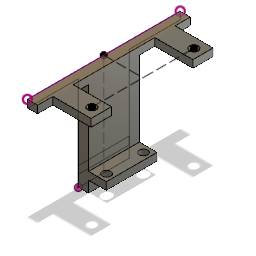
support_carte_front (Autodesk Fusion 360 design; units mm, degrees)
Autodesk Fusion 360 part; units mm, degrees
sketch "Sketch1" plane through (0, 0, 0) normal (1, 0, 0) x (0, 0, -1)
  line L0 (0, 0) -> (0, 37)
  line L1 (0, 37) -> (-20, 37)
  line L2 (-20, 37) -> (-20, 40)
  line L3 (-20, 40) -> (40, 40)
  line L4 (40, 40) -> (40, 37)
  line L5 (40, 37) -> (20, 37)
  line L6 (20, 37) -> (20, 0)
  line L7 (20, 0) -> (0, 0)
  line L8 (0, 4.5) -> (20, 4.5)
  line L9 (20, 4.5) -> (20, 7.5)
  line L10 (20, 7.5) -> (0, 7.5)
  line L11 (0, 7.5) -> (0, 4.5)
  line L12 (10, 0) -> (10, 40) construction
  point P0 (10, 40)
  dimension "d1" = 20
  dimension "d2" = 4.5
  dimension "d3" = 3
  dimension "d5" = 40
  dimension "d7" = 3
  dimension "d8" = 60
  constraint coincident L0.start L7.end
  constraint vertical L0
  constraint perpendicular L0 L1
  constraint perpendicular L1 L2
  constraint perpendicular L2 L3
  constraint perpendicular L3 L4
  constraint perpendicular L4 L5
  constraint perpendicular L3 L6
  constraint perpendicular L0 L7
  constraint horizontal L8
  constraint vertical L9
  constraint horizontal L10
  constraint vertical L11
  constraint coincident L6 L9.end
  constraint coincident L0 L8.start
  constraint collinear L1 L5
  constraint midpoint L3 P0
  constraint midpoint L7 L12.start
  constraint coincident L3 P0
  constraint perpendicular L3 L12
  constraint coincident P0 L12.end
  measures "d1" distance of L0 L6
  measures "d2" distance of L7 L8
  measures "d3" distance of L8 L10
  measures "d5" distance of L3 L7
  measures "d7" distance of L3 L5
  measures "d8" distance of L2 L4
  measures "d23" distance of L0.start
extrude "Extrude1" add sketch "Sketch1" along normal blind 4 makes body 1
extrude "Extrude2" add sketch "Sketch1" along normal blind 11 separate body contours L0 L6 L8 L9 L10 L11 makes body 2
sketch "Sketch2" plane through (0, 7.5, 0) normal (0, 1, 0) x (-1, 0, 0)
  line L0 (0, -20) -> (0, 0)
  line L1 (0, 0) -> (-11, 0)
  line L2 (-11, 0) -> (-11, -20)
  line L3 (-11, -20) -> (0, -20)
  circle A0 centre (-8.35, -17.25) radius 1.65
  circle A1 centre (-8.35, -2.75) radius 1.65
  line L4 (-8.35, -2.75) -> (-8.35, -17.25) construction
  line L5 (-11, -10) -> (-5.7, -10) construction
  point P0 (-8.35, -10)
  dimension "d15" = 14.5
  dimension "d16" = 2.65
  dimension "d17" = 3.3
  dimension "d18" = 3.3
  constraint coincident A1.centre L4.start
  constraint coincident A0.centre L4.end
  constraint parallel L0 L4
  constraint midpoint L2 L5.start
  constraint perpendicular L2 L5
  constraint midpoint L4 P0
  constraint midpoint L5 P0
  measures "d15" distance of A0.centre A1.centre
  measures "d16" distance of L2 L4
  measures "d17" diameter of A1
  measures "d18" diameter of A0
extrude "Extrude3" cut sketch "Sketch2" against normal through all contours A0 | A1 bodies 2
sketch "Sketch3" plane through (0, 40, 0) normal (0, 1, 0) x (-1, 0, 0)
  line L0 (0, -40) -> (0, 20)
  line L1 (0, 20) -> (-4, 20)
  line L2 (-4, 20) -> (-4, -40)
  line L3 (-4, -40) -> (0, -40)
sketch "Sketch4" plane through (0, 40, 0) normal (0, 1, 0) x (-1, 0, 0)
  circle A0 centre (-15.35, -30) radius 1.65
  circle A1 centre (-15.35, 10) radius 1.65
  line L0 (-15.35, 10) -> (-15.35, -30) construction
  line L1 (0, 20) -> (0, -40)
  line L2 (0, -10) -> (-15.35, -10) construction
  dimension "d20" = 40
  dimension "d21" = 3.3
  dimension "d22" = 3.3
  dimension "d23" = 15.35
  constraint vertical L0
  constraint coincident A0.centre L0.end
  constraint coincident A1.centre L0.start
  constraint midpoint L1 L2.start
  constraint perpendicular L1 L2
  constraint coincident L0 L2.end
  constraint midpoint L0 L2.end
  measures "d20" distance of A1.centre A0.centre
  measures "d21" diameter of A1
  measures "d22" diameter of A0
  measures "d23" distance of L0 L1
sketch "Sketch5" plane through (4, 0, 0) normal (1, 0, 0) x (0, 0, -1)
  line L0 (0, 37) -> (0, 0)
  line L1 (0, 0) -> (20, 0)
  line L2 (20, 0) -> (20, 37)
  line L3 (20, 37) -> (40, 37)
  line L4 (40, 37) -> (40, 40)
  line L5 (40, 40) -> (-20, 40)
  line L6 (-20, 40) -> (-20, 37)
  line L7 (-20, 37) -> (0, 37)
  line L8 (-14, 40) -> (-6, 40)
  line L9 (-6, 40) -> (-6, 37)
  line L10 (-6, 37) -> (-14, 37)
  line L11 (-14, 37) -> (-14, 40)
  line L12 (26, 40) -> (34, 40)
  line L13 (34, 40) -> (34, 37)
  line L14 (34, 37) -> (26, 37)
  line L15 (26, 37) -> (26, 40)
  point P0 (-10, 40)
  point P1 (30, 40)
  dimension "d24" = 8
  dimension "d25" = 8
  dimension "d26" = 4
  dimension "d27" = 4
  constraint horizontal L8
  constraint vertical L9
  constraint horizontal L10
  constraint vertical L11
  constraint coincident L7 L9.end
  constraint coincident L5 L8.start
  constraint horizontal L12
  constraint vertical L13
  constraint horizontal L14
  constraint vertical L15
  constraint coincident L3 L13.end
  constraint coincident L5 L12.start
  measures "d24" distance of L13 L15
  measures "d25" distance of L9 L11
  measures "d26" distance of L11 P0
  measures "d27" distance of L15 P1
extrude "Extrude4" add sketch "Sketch5" along normal blind 15 contours L5 L7 L8 L9 L10 L11 | L3 L5 L12 L13 L14 L15 bodies 1
extrude "Extrude5" cut sketch "Sketch4" against normal through all bodies 1
combine "Combine1" operation add target body 2 tool bodies 1
equation "d3 = e"
equation "e = 3 mm"
equation "d7 = e"
equation "t = 3.3 mm"
equation "d16 = 1 mm + ( 3.3 / 2 ) * 1 mm"
equation "d17 = t"
equation "d18 = t"
equation "d21 = t"
equation "d22 = t"
